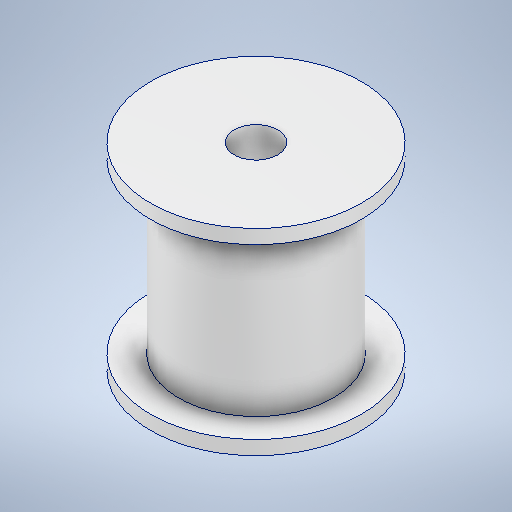
# Autodesk Inventor part: poulie courroie
Saved by Autodesk Inventor 2025.1 (Build 291241000, 241)
## iProperties
Created: 2025-03-24
Part Number: poulie courroie
Material: Générique
Document SubType Name: Modeling
Designer: felix
Density: 1 g/cm^3
Appearance: Aluminium - Plat
Author: felix
Autodesk Inventor part; units mm, degrees
ref_plane "YZ Plane" through (0, 0, 0) normal (1, 0, 0) x (0, 1, 0)
ref_plane "XZ Plane" through (0, 0, 0) normal (0, 1, 0) x (-1, 0, 0)
ref_plane "XY Plane" through (0, 0, 0) normal (0, 0, 1) x (1, 0, 0)
sketch "Esquisse2" plane through (0, 0, 0) normal (0, 0, 1) x (1, 0, 0)
  line L0 (0, 17.0922) -> (0, -5.3775) construction
  line L1 (0, 0) -> (7.5, 0)
  line L2 (7.5, 0) -> (7.5, 1)
  line L3 (7.5, 1) -> (5.5, 1)
  line L4 (5.5, 1) -> (5.5, 13)
  line L5 (5.5, 13) -> (7.5, 13)
  line L6 (7.5, 13) -> (7.5, 14)
  line L7 (7.5, 14) -> (0, 14)
  line L8 (0, 14) -> (0, 0)
  dimension "d8" = 15
  dimension "d9" = 1
  dimension "d10" = 1
  dimension "d11" = 14
  dimension "d12" = 2
  dimension "d20" = 7.5
  constraints: 18 end point, 6 perpendicular, 1 collinear, 1 horizontal, 1 point on line, 1 vertical
  measures "d8" diameter of L6 L0
  measures "d9" distance of L5.end L6.end
  measures "d10" distance of L1.end L2.end
  measures "d11" distance between parallel lines of L1 L7
  measures "d12" distance of L4.end L5.end
  measures "d20" distance of L1.start L1.end
revolve "Révolution1" add sketch "Esquisse2" angle 360 about axis through (0, 17.0922, 0) along (0, -1, 0)
sketch "Esquisse3" plane through (0, 14, 0) normal (0, 1, 0) x (1, 0, 0)
  point P0 (0, 0)
  point P1 (0, 0)
  constraints: 1 coincident
hole "Perçage1" at (0, 14, 0) direction (0, -1, 0) diameter 3.1 end through all clearance for "Vis d'assemblage à six pans creux" size "M3" standard "Profil M métrique ANSI"
equation "\"d20\" = 0.5 * d8"
